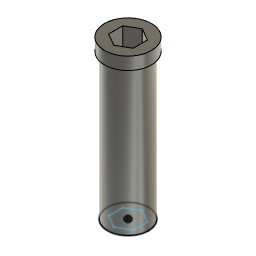
fineline-mount-pen-holder (Autodesk Fusion 360 design; units mm, degrees)
Autodesk Fusion 360 part; units mm, degrees
sketch "Sketch1" plane through (0, 0, 0) normal (0, 0, 1) x (1, 0, 0)
  circle A0 centre (0, 0) radius 6.5
  line L0 (0.0017, 4.55) -> (-3.9396, 2.2765)
  line L1 (-3.9396, 2.2765) -> (-3.9413, -2.2735)
  line L2 (-3.9413, -2.2735) -> (-0.0017, -4.55)
  line L3 (-0.0017, -4.55) -> (3.9396, -2.2765)
  line L4 (3.9396, -2.2765) -> (3.9413, 2.2735)
  line L5 (3.9413, 2.2735) -> (0.0017, 4.55)
  circle A1 centre (0, 0) radius 1
  dimension "d1" = 13
  dimension "d2" = 4.55
  dimension "d3" = 2
  constraint coincident A0.centre A1.centre
  constraint concentric A0 A1
  measures "d1" diameter of A0
  measures "d2" distance of L0.start A0.centre
  measures "d3" diameter of A1
extrude "Extrude1" add sketch "Sketch1" along normal blind 46.4 contours A0
extrude "Extrude2" add sketch "Sketch1" along normal blind 1 contours L0 L1 L2 L3 L4 L5
sketch "Sketch2" plane through (0, 0, 1) normal (0, 0, 1) x (-1, 0, 0)
  circle A0 centre (0, 0) radius 1
  line L0 (-3.9413, -2.2735) -> (-0.0017, -4.55)
  line L1 (-0.0017, -4.55) -> (3.9396, -2.2765)
  line L2 (3.9396, -2.2765) -> (3.9413, 2.2735)
  line L3 (3.9413, 2.2735) -> (0.0017, 4.55)
  line L4 (0.0017, 4.55) -> (-3.9396, 2.2765)
  line L5 (-3.9396, 2.2765) -> (-3.9413, -2.2735)
  circle A1 centre (0, 0) radius 5
  dimension "d8" = 10
  constraint coincident A0.centre A1.centre
  measures "d8" diameter of A1
extrude "Extrude3" cut sketch "Sketch2" along normal blind 25 contours A1
chamfer "Chamfer1" distance 0.5 distance2 1 1 edges at (4.6616, 1.8081, 26) measured on face at (-4.9752, 0.4978, 9.3333)
sketch "Sketch3" plane through (0, 0, 46.4) normal (0, 0, 1) x (-1, 0, 0)
  line L0 (-0.0017, -4.55) -> (-3.9413, -2.2735)
  line L1 (-3.9413, -2.2735) -> (-3.9396, 2.2765)
  line L2 (-3.9396, 2.2765) -> (0.0017, 4.55)
  line L3 (0.0017, 4.55) -> (3.9413, 2.2735)
  line L4 (3.9413, 2.2735) -> (3.9396, -2.2765)
  line L5 (3.9396, -2.2765) -> (-0.0017, -4.55)
  circle A0 centre (0, 0) radius 6.5
  circle A1 centre (0, 0) radius 7.5
  dimension "d13" = 15
  constraint concentric A0 A1
  measures "d13" diameter of A1
extrude "Extrude4" add sketch "Sketch3" along normal blind 4 contours A0 | A1
